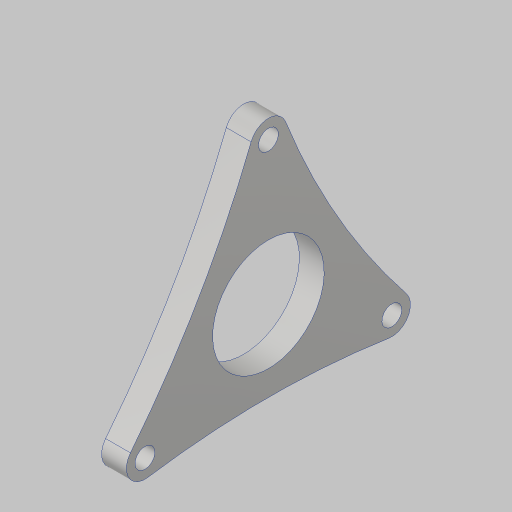
# Autodesk Inventor part: AR-004
Saved by Autodesk Inventor 2023.5 (Build 275446000, 446)
## iProperties
Created: 2025-01-22
Part Number: AR-004
Material: Aluminum 6061
Document SubType Name: Modeling
Designer: slick
Density: 2.7 g/cm^3
Appearance: Aluminum - Flat
Author: slick
Autodesk Inventor part; units mm, degrees
ref_plane "YZ Plane" through (0, 0, 0) normal (1, 0, 0) x (0, 1, 0)
ref_plane "XZ Plane" through (0, 0, 0) normal (0, 1, 0) x (-1, 0, 0)
ref_plane "XY Plane" through (0, 0, 0) normal (0, 0, 1) x (1, 0, 0)
sketch "Sketch1" plane through (0, 0, 0) normal (1, 0, 0) x (0, 1, 0)
  circle A0 centre (0, 0) radius 31.75 construction
  circle A1 centre (36.5125, 0) radius 4.7625 construction
  circle A2 centre (-18.2562, 31.6208) radius 4.7625 construction
  circle A3 centre (-18.2563, -31.6208) radius 4.7625 construction
  circle A4 centre (0, 0) radius 14.2875
  circle A5 centre (0, 0) radius 20.6375 construction
  arc A6 (-15.2842, 35.3421) -> (38.2492, 4.4346) centre (113.5062, 196.5986) ccw
  arc A7 (38.2492, -4.4346) -> (-15.2842, -35.3421) centre (113.5062, -196.5986) ccw
  arc A8 (-22.965, -30.9075) -> (-22.965, 30.9075) centre (-227.0125, 0) ccw
  arc A9 (38.2492, -4.4346) -> (38.2492, 4.4346) centre (36.5125, 0) ccw
  arc A10 (-22.965, -30.9075) -> (-15.2842, -35.3421) centre (-18.2563, -31.6208) ccw
  arc A11 (-15.2842, 35.3421) -> (-22.965, 30.9075) centre (-18.2562, 31.6208) ccw
  dimension "d0" = 63.5
  dimension "d1" = 9.525
  dimension "d4" = 360
  dimension "d6" = 28.575
  dimension "d7" = 6.35
  constraints: 18 point on circle, 12 centre point, 10 tangent, 8 coincident, 1 concentric, 1 horizontal alignment, 7 other
  measures "d0" diameter of A0
  measures "d1" diameter of A1
  measures "d6" diameter of A4
  measures "d7" radial gap between concentric circles of A4 A5
extrude "Extrusion1" add sketch "Sketch1" along normal blind 6.35
hole "Hole1" at (0, 36.5125, 0) at (0, -18.2562, 31.6208) at (0, -18.2563, -31.6208) direction (1, 0, 0) diameter 5.1054 end through all clearance for "Flat Head Machine Screw (82)" size "#10" standard "Ansi Unified Screw Threads"
body "Solid1"
